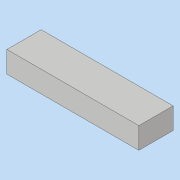
# Autodesk Inventor part: lw_6_part1
Saved by Autodesk Inventor 2019 (Build 230136000, 136)
## iProperties
Created: 2021-05-14
Part Number: lw_6_part1
Material: Типовые
Document SubType Name: Modeling
Designer: Kurbatova
Density: 1 g/cm^3
Appearance: По умолчанию
parametr_A_: 185,000 мм
parametr_B_: 48,000 мм
Author: Kurbatova
Autodesk Inventor part; units mm, degrees
ref_plane "YZ Plane" through (0, 0, 0) normal (1, 0, 0) x (0, 1, 0)
ref_plane "XZ Plane" through (0, 0, 0) normal (0, 1, 0) x (-1, 0, 0)
ref_plane "XY Plane" through (0, 0, 0) normal (0, 0, 1) x (1, 0, 0)
sketch "Эскиз1" plane through (0, 0, 0) normal (0, 0, 1) x (1, 0, 0)
  line L0 (-88.1763, -30) -> (96.8237, -30)
  line L1 (-88.1763, -30) -> (-88.1763, 0)
  line L2 (96.8237, 0) -> (96.8237, -30)
  line L3 (-88.1763, 0) -> (96.8237, 0)
  point P0 (0, 0)
  point P1 (0, -30)
  dimension "parametr_A" = 185
  dimension "parametr_C" = 30
  constraints: 8 end point, 2 horizontal, 1 point on line, 1 vertical
  measures "parametr_A" distance of L0.start L0.end
  measures "parametr_C" distance of L1.end L0.start
extrude "Выдавливание2" add sketch "Эскиз1" along normal blind 48
equation "\"parametr_A\" = parametr_A_"
equation "\"paramert_B\" = parametr_B_"
equation "\"parametr_A_\" = 185"
equation "\"parametr_B_\" = 48"
